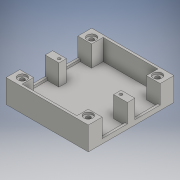
# Autodesk Inventor part: NUCBasePCB
Saved by Autodesk Inventor 2016 (Build 200138000, 138)
## iProperties
Created: 2015-09-23
Part Number: NUCBasePCB
Material: Generic
Document SubType Name: Modeling
Designer: lachesis
Density: 1 g/cm^3
Appearance: Default
Author: lachesis
Autodesk Inventor part; units mm, degrees
ref_plane "YZ Plane" through (0, 0, 0) normal (1, 0, 0) x (0, 1, 0)
ref_plane "XZ Plane" through (0, 0, 0) normal (0, 1, 0) x (-1, 0, 0)
ref_plane "XY Plane" through (0, 0, 0) normal (0, 0, 1) x (1, 0, 0)
sketch "Sketch1" plane through (0, 0, 0) normal (0, 1, 0) x (-1, 0, 0)
  line L0 (58.42, 56.134) -> (-58.42, 56.134)
  line L1 (-58.42, 56.134) -> (-58.42, -56.134)
  line L2 (-58.42, -56.134) -> (58.42, -56.134)
  line L3 (58.42, -56.134) -> (58.42, 56.134)
  point P0 (0, 0)
  point P1 (0, -56.134)
  point P2 (58.42, 0)
  dimension "d0" = 112.268
  dimension "d1" = 116.84
  constraints: 8 end point, 2 midpoint, 2 parallel, 1 horizontal, 1 horizontal alignment, 1 perpendicular, 1 vertical alignment
  measures "d0" distance of L2.end L0.start
  measures "d1" distance of L1.end L2.end
extrude "Extrusion1" add sketch "Sketch1" along normal blind 31.75
sketch "Sketch2" plane through (0, 31.75, 0) normal (0, 1, 0) x (1, 0, 0)
  line L0 (58.42, -56.134) -> (58.42, 56.134) projected
  line L1 (58.42, 56.134) -> (-58.42, 56.134) projected
  line L2 (-58.42, -56.134) -> (58.42, -56.134) projected
  line L3 (-58.42, 56.134) -> (-58.42, -56.134) projected
  point P0 (0, 0)
  point P1 (47.244, 44.958)
  point P2 (47.244, -44.958)
  point P3 (-47.244, 44.958)
  point P4 (-47.244, -44.958)
  dimension "d4" = 11.176
  dimension "d5" = 11.176
  dimension "d6" = 11.176
  dimension "d7" = 11.176
  constraints: 2 horizontal alignment, 2 vertical alignment
  measures "d4" distance from line of L0 point (47.244, 44.958)
  measures "d5" distance from line of L1 point (47.244, 44.958)
  measures "d6" distance from line of L2 point (-47.244, -44.958)
  measures "d7" distance from line of L3 point (-47.244, -44.958)
hole "Hole1" at (47.244, 31.75, -44.958) at (47.244, 31.75, 44.958) at (-47.244, 31.75, -44.958) at (-47.244, 31.75, 44.958) direction (0, -1, 0) diameter 3.302 end through all counterbore diameter 5.969 counterbore depth 26.162
sketch "Sketch3" plane through (0, 31.75, 0) normal (0, 1, 0) x (1, 0, 0)
  circle A0 centre (47.244, 44.958) radius 2.9845 projected
  circle A1 centre (47.244, -44.958) radius 2.9845 projected
  circle A2 centre (-47.244, 44.958) radius 2.9845 projected
  circle A3 centre (-47.244, -44.958) radius 2.9845 projected
  circle A4 centre (47.244, 44.958) radius 1.651 projected
  circle A5 centre (47.244, -44.958) radius 1.651 projected
  circle A6 centre (-47.244, -44.958) radius 1.651 projected
  point P0 (0, 0)
  constraints: 4 coincident
hole "Hole2" at (47.244, 31.75, -44.958) at (47.244, 31.75, 44.958) at (-47.244, 31.75, 44.958) at (-47.244, 31.75, -44.958) direction (0, -1, 0) diameter 12.065 depth 2.413
sketch "Sketch5" plane through (0, 0, 0) normal (0, -1, 0) x (1, 0, 0)
  circle A0 centre (-47.244, 44.958) radius 1.651 projected
  circle A1 centre (-47.244, -44.958) radius 1.651 projected
  point P0 (0, 0)
  point P1 (0, 42.164)
  point P2 (0, -42.164)
  dimension "d25" = 47.244
  dimension "d26" = 2.794
  dimension "d27" = 2.794
  constraints: 1 vertical alignment
  measures "d25" horizontal distance of A0.centre point (0, 42.164)
  measures "d26" vertical distance of A0.centre point (0, 42.164)
  measures "d27" vertical distance of A1.centre point (0, -42.164)
hole "Hole3" at (0, 0, 42.164) at (0, 0, -42.164) direction (0, 1, 0) diameter 3.9116 end through all counterbore diameter 6.604 counterbore depth 19.558
sketch "Sketch6" plane through (0, 31.75, 0) normal (0, 1, 0) x (1, 0, 0)
  circle A0 centre (0, -42.164) radius 1.9558 projected
  circle A1 centre (0, 42.164) radius 1.9558 projected
  circle A2 centre (-47.244, -44.958) radius 6.0325 projected
  circle A3 centre (47.244, 44.958) radius 6.0325 projected
  circle A4 centre (47.244, -44.958) radius 6.0325 projected
  circle A5 centre (-47.244, 44.958) radius 6.0325 projected
  line L0 (-58.42, -56.134) -> (58.42, -56.134) projected
  line L1 (58.42, -56.134) -> (58.42, 56.134) projected
  line L2 (58.42, 56.134) -> (-58.42, 56.134) projected
  line L3 (-58.42, 56.134) -> (-58.42, -56.134) projected
  line L4 (39.624, 52.959) -> (39.624, 37.338)
  line L5 (39.624, 37.338) -> (55.245, 37.338)
  line L6 (55.245, 37.338) -> (55.245, -37.338)
  line L7 (55.245, -37.338) -> (39.624, -37.338)
  line L8 (39.624, -37.338) -> (39.624, -52.959)
  line L9 (-39.624, -52.959) -> (-39.624, -37.338)
  line L10 (-39.624, -37.338) -> (-55.245, -37.338)
  line L11 (-55.245, -37.338) -> (-55.245, 37.338)
  line L12 (-55.245, 37.338) -> (-39.624, 37.338)
  line L13 (-39.624, 37.338) -> (-39.624, 52.959)
  line L14 (-39.624, -52.959) -> (-5.08, -52.959)
  line L15 (-5.08, -52.959) -> (-5.08, -37.338)
  line L16 (-5.08, -37.338) -> (5.08, -37.338)
  line L17 (5.08, -37.338) -> (5.08, -52.959)
  line L18 (5.08, -52.959) -> (39.624, -52.959)
  line L19 (-39.624, 52.959) -> (-5.08, 52.959)
  line L20 (-5.08, 52.959) -> (-5.08, 37.338)
  line L21 (-5.08, 37.338) -> (5.08, 37.338)
  line L22 (5.08, 37.338) -> (5.08, 52.959)
  line L23 (5.08, 52.959) -> (39.624, 52.959)
  point P0 (0, 0)
  dimension "d36" = 3.175
  dimension "d37" = 15.621
  dimension "d38" = 15.621
  dimension "d39" = 15.621
  dimension "d41" = 3.175
  dimension "d42" = 5.08
  dimension "d43" = 5.08
  dimension "d44" = 3.175
  dimension "d45" = 3.175
  constraints: 40 end point, 15 perpendicular, 7 equal length, 3 point on line, 2 horizontal, 1 collinear, 1 vertical
  measures "d36" distance between parallel lines of L3 L11
  measures "d37" distance of L12.end L13.end
  measures "d38" distance of L7.end L8.end
  measures "d39" distance of L9.end L10.end
  measures "d41" distance between parallel lines of L1 L6
  measures "d42" distance from line of A0.centre L17
  measures "d43" distance from line of A0.centre L15
  measures "d44" distance between parallel lines of L0 L14
  measures "d45" distance between parallel lines of L2 L19
extrude "Extrusion2" cut sketch "Sketch6" against normal blind 28.575 contours L4 L5 L6 L7 L8 L18 L17 L16 L15 L14 L9 L10 L11 L12 L13 L19 L20 L21 L22 L23
sketch "Sketch7" plane through (-58.42, 0, 56.134) normal (0, 0, 1) x (1, 0, 0)
  line L0 (0, 0) -> (116.84, 0) projected
  line L1 (116.84, 0) -> (116.84, 31.75) projected
  line L2 (0, 31.75) -> (116.84, 31.75) projected
  line L3 (0, 0) -> (0, 31.75) projected
  line L4 (53.34, 3.175) -> (18.796, 3.175) projected
  line L5 (98.044, 3.175) -> (63.5, 3.175) projected
  line L6 (98.044, 31.75) -> (98.044, 3.175) projected
  line L7 (18.796, 31.75) -> (18.796, 3.175) projected
  line L8 (63.5, 31.75) -> (63.5, 3.175) projected
  line L9 (53.34, 31.75) -> (53.34, 3.175) projected
  line L10 (18.796, 31.75) -> (18.796, 3.175) projected
  line L11 (53.34, 31.75) -> (53.34, 3.175) projected
  line L12 (18.796, 31.75) -> (53.34, 31.75)
  line L13 (53.34, 31.75) -> (53.34, 6.35)
  line L14 (53.34, 6.35) -> (18.796, 6.35)
  line L15 (18.796, 6.35) -> (18.796, 31.75)
  line L16 (63.5, 31.75) -> (98.044, 31.75) projected
  line L17 (63.5, 31.75) -> (98.044, 31.75)
  line L18 (98.044, 31.75) -> (98.044, 6.35)
  line L19 (98.044, 6.35) -> (63.5, 6.35)
  line L20 (63.5, 6.35) -> (63.5, 31.75)
  point P0 (58.42, 0)
  dimension "d48" = 3.175
  constraints: 16 end point, 4 parallel, 2 horizontal, 2 perpendicular, 2 point on line, 1 collinear
  measures "d48" distance between parallel lines of L4 L14
extrude "Extrusion3" cut sketch "Sketch7" against normal through all contours L2 L9 L14 L7 | L6 L19 L8 L2
equation "\"d5\" = d4"
equation "\"d6\" = d4"
equation "\"d7\" = d4"
equation "\"d38\" = d37"
equation "\"d39\" = d37"
equation "\"d41\" = d36"
equation "\"d43\" = d42"
equation "\"d44\" = d36"
equation "\"d45\" = d36"
body "Solid1"
